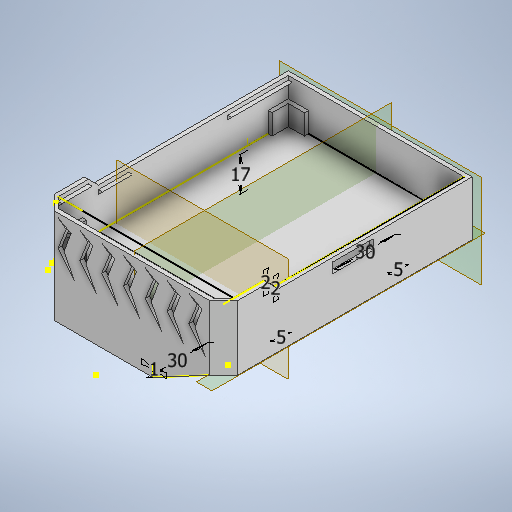
# Autodesk Inventor part: Part1edd
Saved by Autodesk Inventor 2025.2 (Build 292293000, 293)
## iProperties
Created: 2025-06-04
Part Number: Part1edd
Material: Generic
Document SubType Name: Sheet Metal
Designer: ziyuz
Density: 1 g/cm^3
Sheet Metal Rule: Default_mm
Appearance: Default
Author: ziyuz
Autodesk Inventor part; units mm, degrees
ref_plane "YZ Plane" through (0, 0, 0) normal (1, 0, 0) x (0, 1, 0)
ref_plane "XZ Plane" through (0, 0, 0) normal (0, 1, 0) x (-1, 0, 0)
ref_plane "XY Plane" through (0, 0, 0) normal (0, 0, 1) x (1, 0, 0)
sketch "Sketch1" plane through (0, 0, 0) normal (0, 1, 0) x (-1, 0, 0)
  line L0 (0, 0) -> (-85, 0)
  line L1 (-85, 0) -> (-85, -115)
  line L2 (-85, -115) -> (0, -115)
  line L3 (0, -115) -> (0, 0)
  dimension "d0" = 85
  dimension "d1" = 115
  constraints: 8 end point, 2 parallel, 1 horizontal, 1 perpendicular
  measures "d0" distance of L2.end L1.end
  measures "d1" distance of L1.end L0.end
extrude "Extrusion1" add sketch "Sketch1" along normal blind 2
sketch "Sketch2" plane through (0, 2, 0) normal (0, 1, 0) x (1, 0, 0)
  line L0 (0, 115) -> (0, 0) projected
  line L1 (0, 115) -> (-2, 115)
  line L2 (0, 115) -> (0, 117)
  line L3 (0, 117) -> (-2, 117)
  line L4 (-2, 115) -> (-2, 117)
  line L5 (-2, 117) -> (87, 117)
  line L6 (87, 117) -> (87, -2)
  line L7 (87, -2) -> (-2, -2)
  line L8 (-2, -2) -> (-2, 117)
  line L9 (-2, 117) -> (-2, 107)
  line L10 (-2, 107) -> (0, 107)
  line L11 (-2, 117) -> (8, 117)
  line L12 (8, 117) -> (8, 115)
  line L13 (85, 115) -> (0, 115) projected
  line L14 (-2, 115) -> (-2, 5)
  line L15 (-2, 5) -> (-2, 15)
  line L16 (0, 15) -> (0, 5)
  line L17 (8, 5) -> (8, 7)
  line L18 (-2, 5) -> (-2, 3)
  line L19 (-2, 3) -> (10, 3)
  line L20 (10, 3) -> (10, 5)
  line L21 (10, 5) -> (0, 5)
  line L22 (0, 5) -> (0, 15)
  line L23 (0, 15) -> (-2, 15)
  line L24 (-2, 5) -> (-2, 15)
  dimension "d4" = 2
  dimension "d5" = 2
  dimension "d6" = 89
  dimension "d7" = 119
  dimension "d8" = 10
  dimension "d9" = 10
  dimension "d10" = 110
  dimension "d11" = 10
  dimension "d13" = 2
  dimension "d21" = 2
  dimension "d22" = 12
  dimension "d23" = 2
  dimension "d24" = 10
  constraints: 46 end point, 9 point on line, 7 perpendicular, 3 parallel, 2 collinear, 2 horizontal, 1 vertical
  measures "d4" distance of L0.start L1.end
  measures "d5" distance of L0.start L2.end
  measures "d6" distance of L6.end L7.end
  measures "d7" distance of L5.end L6.end
  measures "d8" distance of L3.end L9.end
  measures "d9" distance of L3.end L11.end
  measures "d10" distance of L1.end L14.end
  measures "d11" distance of L14.end L15.end
  measures "d13" distance of L17.start L17.end
  measures "d21" distance of L14.end L18.end
  measures "d22" distance of L18.end L19.end
  measures "d23" distance of L19.end L20.end
  measures "d24" distance of L16.end L16.start
extrude "Extrusion2" add sketch "Sketch2" along normal blind 10 contours L0 L10 L8 L1 | L1 L4 L3 L2 | L2 L5 L12 L13 | L0 L19 L8 L23 | L21 L20 L19 L0
sketch "Sketch3" plane through (0, 2, 0) normal (0, -1, 0) x (1, 0, 0)
  line L0 (8, -117) -> (-2, -117) projected
  line L1 (-2, -117) -> (85, -117)
  line L2 (85, -117) -> (85, 2)
  line L3 (85, 2) -> (-2, 2)
  line L4 (-2, 2) -> (-2, -117)
  point P0 (0, 0)
  point P1 (87, -117)
  dimension "d16" = 87
  dimension "d17" = 119
  constraints: 8 end point, 2 parallel, 1 horizontal, 1 perpendicular
  measures "d16" distance of L3.end L2.end
  measures "d17" distance of L2.end L1.end
extrude "Extrusion3" add sketch "Sketch3" along normal blind 2
sketch "Sketch5" plane through (0, 2, 0) normal (0, 1, 0) x (1, 0, 0)
  line L0 (0, 5) -> (0, 15) projected
  line L1 (85, 117) -> (85, -2) projected
  line L2 (0, 5) -> (85, 5)
  line L3 (85, 5) -> (85, 115)
  line L4 (85, 115) -> (0, 115)
  line L5 (0, 115) -> (0, 5)
  line L6 (0, 5) -> (40, 5)
  line L7 (85, 5) -> (50, 5)
  line L8 (85, -2) -> (-2, -2) projected
  line L9 (40, 5) -> (50, 5)
  line L10 (50, 5) -> (50, -2)
  line L11 (50, -2) -> (40, -2)
  line L12 (40, -2) -> (40, 5)
  point P0 (0, 0)
  dimension "d25" = 110
  dimension "d26" = 40
  dimension "d27" = 35
  constraints: 20 end point, 4 parallel, 4 point on line, 2 horizontal, 2 perpendicular
  measures "d25" distance of L3.end L2.end
  measures "d26" distance of L0.start L6.end
  measures "d27" distance of L2.end L7.end
extrude "Extrusion4" cut sketch "Sketch5" against normal blind 10 contours L2 L10 L8 L12
sketch "Sketch6" plane through (0, 0, 0) normal (0, -1, 0) x (1, 0, 0)
  line L0 (-2, 2) -> (-2, -3) projected
  line L1 (-2, 2) -> (-4, 2)
  line L2 (-4, 2) -> (-4, 4)
  line L3 (-4, 4) -> (-2, 4)
  line L4 (-2, 4) -> (-2, 2)
  line L5 (-4, 4) -> (87, 4)
  line L6 (87, 4) -> (87, -119)
  line L7 (87, -119) -> (-4, -119)
  line L8 (-4, -119) -> (-4, 4)
  line L9 (85, -117) -> (85, 2) projected
  line L10 (-2, 2) -> (85, 2)
  line L11 (85, 2) -> (85, -117)
  line L12 (85, -117) -> (-2, -117)
  line L13 (-2, -117) -> (-2, 2)
  line L14 (-2, -3) -> (-4, -3)
  line L15 (-4, -3) -> (-4, 4)
  line L16 (-4, 4) -> (3, 4)
  line L17 (3, 4) -> (3, 2)
  line L18 (-2, -3) -> (3, 2)
  line L19 (85, -3) -> (85, 2)
  line L20 (85, 2) -> (80, 2)
  line L21 (80, 2) -> (85, -3)
  line L22 (87, -3) -> (85, -3)
  line L23 (80, 2) -> (80, 4)
  line L24 (-4, -3) -> (3, 4)
  line L25 (3, 2) -> (-2, -3)
  line L26 (87, -3) -> (80, 4)
  point P0 (0, 0)
  point P1 (85, 2)
  point P2 (-2, -3)
  point P3 (-2, -3)
  dimension "d30" = 2
  dimension "d31" = 2
  dimension "d32" = 91
  dimension "d33" = 123
  dimension "d36" = 7
  dimension "d37" = 5
  constraints: 50 end point, 8 point on line, 7 parallel, 6 perpendicular, 3 horizontal, 2 collinear
  measures "d30" distance of L2.end L3.end
  measures "d31" distance of L1.end L2.end
  measures "d32" distance of L6.end L7.end
  measures "d33" distance of L5.end L6.end
  measures "d36" distance of L2.end L16.end
  measures "d37" distance of L10.end L20.end
extrude "Extrusion5" add sketch "Sketch6" against normal blind 22 contours L24 L10 L18 L0 | L0 L14 L24 | L24 L17 L10 | L13 L12 L9 L22 L6 L7 L8 L14 | L5 L23 L10 L17 | L26 L10 L23 | L10 L26 L9 L21 | L9 L26 L22
sketch "Sketch7" plane through (0, 2, 0) normal (0, 1, 0) x (1, 0, 0)
  line L0 (-2, -2) -> (-2, 1) projected
  line L1 (-2, -2) -> (-2, 1)
  line L2 (1, -2) -> (-2, -2) projected
  line L3 (1, -2) -> (-2, 1)
  line L4 (-2, -2) -> (1, -2)
  line L5 (85, 1) -> (85, -2) projected
  line L6 (85, -2) -> (85, 1)
  line L7 (85, -2) -> (82, -2)
  line L8 (80, -4) -> (87, 3) projected
  line L9 (85, 1) -> (82, -2)
  point P0 (0, 0)
  constraints: 12 end point, 2 collinear, 2 point on line, 2 vertical
extrude "Extrusion6" cut sketch "Sketch7" against normal blind 22
sketch "Sketch8" plane through (0, 22, 0) normal (0, 1, 0) x (1, 0, 0)
  line L0 (-4, 3) -> (-4, 23)
  line L1 (-4, 3) -> (-4, 119) projected
  line L2 (-4, 23) -> (-2, 23)
  line L3 (-2, 3) -> (-2, 117) projected
  line L4 (-2, 3) -> (3, -2) projected
  line L5 (-2, 3) -> (3, -2)
  line L6 (85, 3) -> (80, -2) projected
  line L7 (3, -2) -> (80, -2)
  line L8 (80, -2) -> (85, 3)
  line L9 (85, 117) -> (85, 3) projected
  line L10 (85, 3) -> (85, 23)
  line L11 (85, 23) -> (87, 23)
  line L12 (87, 119) -> (87, 3) projected
  line L13 (80, -4) -> (87, 3) projected
  line L14 (87, 3) -> (87, 23)
  line L15 (87, 3) -> (80, -4)
  line L16 (-4, 3) -> (3, -4) projected
  line L17 (80, -4) -> (3, -4)
  line L18 (3, -4) -> (-4, 3)
  point P0 (0, 0)
  dimension "d40" = 20
  dimension "d41" = 20
  constraints: 22 end point, 5 point on line, 3 collinear, 2 parallel, 2 perpendicular
  measures "d40" distance of L0.start L0.end
  measures "d41" distance of L6.start L10.end
extrude "Extrusion7" add sketch "Sketch8" along normal blind 5
chamfer "Chamfer1" distance 5 angle 45 2 edges at (86, 27, -23) (-3, 27, -23)
sketch "Sketch9" plane through (3, 0, 4) normal (0, 0, 1) x (1, 0, 0)
  line L0 (0, 2) -> (0, 27) projected
  line L1 (0, 27) -> (0, 25)
  line L2 (0, 2) -> (0, 25)
  line L3 (0, 25) -> (77, 25)
  line L4 (0, 27) -> (77, 27) projected
  line L5 (77, 2) -> (77, 27) projected
  line L6 (77, 25) -> (77, 2)
  line L7 (0, 2) -> (77, 2)
  line L8 (0, 2) -> (2, 2)
  line L9 (5, 2) -> (-3, 2) projected
  line L10 (2, 2) -> (2, 25)
  line L11 (77, 25) -> (75, 25)
  line L12 (75, 25) -> (75, 2)
  line L13 (2, 25) -> (6, 22)
  line L14 (-5, 22) -> (82, 22) projected
  line L15 (6, 22) -> (2, 12)
  line L16 (7, 12) -> (-3, 12) projected
  line L17 (0, 2) -> (10, 2)
  line L18 (5, 2) -> (82, 2) projected
  line L19 (10, 2) -> (10, 25)
  line L20 (2, 12) -> (10, 2)
  line L21 (10, 2) -> (5, 12)
  line L22 (5, 12) -> (8.4202, 21.3969)
  line L23 (5, 12) -> (15, 12) construction
  line L24 (2, 25) -> (8.4202, 21.3969)
  line L25 (12.8, 12) -> (20.8, 2)
  line L26 (20.8, 2) -> (15.8, 12)
  line L27 (15.8, 12) -> (19.2202, 21.3969)
  line L28 (16.8, 22) -> (12.8, 12)
  line L29 (12.8, 25) -> (16.8, 22)
  line L30 (12.8, 25) -> (19.2202, 21.3969)
  line L31 (23.6, 12) -> (31.6, 2)
  line L32 (31.6, 2) -> (26.6, 12)
  line L33 (26.6, 12) -> (30.0202, 21.3969)
  line L34 (27.6, 22) -> (23.6, 12)
  line L35 (23.6, 25) -> (27.6, 22)
  line L36 (23.6, 25) -> (30.0202, 21.3969)
  line L37 (34.4, 12) -> (42.4, 2)
  line L38 (42.4, 2) -> (37.4, 12)
  line L39 (37.4, 12) -> (40.8202, 21.3969)
  line L40 (38.4, 22) -> (34.4, 12)
  line L41 (34.4, 25) -> (38.4, 22)
  line L42 (34.4, 25) -> (40.8202, 21.3969)
  line L43 (45.2, 12) -> (53.2, 2)
  line L44 (53.2, 2) -> (48.2, 12)
  line L45 (48.2, 12) -> (51.6202, 21.3969)
  line L46 (49.2, 22) -> (45.2, 12)
  line L47 (45.2, 25) -> (49.2, 22)
  line L48 (45.2, 25) -> (51.6202, 21.3969)
  line L49 (56, 12) -> (64, 2)
  line L50 (64, 2) -> (59, 12)
  line L51 (59, 12) -> (62.4202, 21.3969)
  line L52 (60, 22) -> (56, 12)
  line L53 (56, 25) -> (60, 22)
  line L54 (56, 25) -> (62.4202, 21.3969)
  line L55 (66.8, 12) -> (74.8, 2)
  line L56 (74.8, 2) -> (69.8, 12)
  line L57 (69.8, 12) -> (73.2202, 21.3969)
  line L58 (70.8, 22) -> (66.8, 12)
  line L59 (66.8, 25) -> (70.8, 22)
  line L60 (66.8, 25) -> (73.2202, 21.3969)
  point P0 (-3, 0)
  dimension "d47" = 2
  dimension "d48" = 2
  dimension "d49" = 2
  dimension "d50" = 5
  dimension "d51" = 10
  dimension "d52" = 10
  dimension "d53" = 70
  dimension "d56" = 10.8
  constraints: 108 end point, 9 point on line, 4 perpendicular, 2 collinear, 2 horizontal, 1 equal length, 1 midpoint, 1 parallel, 72 other
  measures "d47" distance of L0.end L1.end
  measures "d48" distance of L0.start L8.end
  measures "d49" distance of L3.end L11.end
  measures "d50" distance of L10.end L13.end
  measures "d51" distance of L0.start L17.end
  measures "d52" distance of L21.end L22.end
  measures "d53" angle of L23 L22
  measures "d56" distance of L15.end L25.start
extrude "Extrusion8" cut sketch "Sketch9" against normal blind 5 contours L24 L14 L13 | L14 L24 L22 L16 L15 | L16 L21 L20 | L30 L14 L29 | L36 L14 L35 | L14 L30 L27 L26 L25 L28 | L60 L14 L59 | L42 L14 L41 | L14 L36 L33 L32 L31 L34 | L54 L14 L53 | L14 L60 L57 L56 L55 L58 | L48 L14 L47 | L14 L42 L39 L38 L37 L40 | L14 L54 L51 L50 L49 L52 | L14 L48 L45 L44 L43 L46
sketch "Sketch10" plane through (87, 0, -3) normal (1, 0, 0) x (0, 0, -1)
  line L0 (112, 2) -> (112, 12) projected
  line L1 (112, 2) -> (2, 2)
  line L2 (114, 12) -> (104, 12) projected
  line L3 (112, 2) -> (222, 2) construction
  line L4 (12, 2) -> (104, 2) projected
  line L5 (0, 0) -> (116, 0) projected
  line L6 (112, 2) -> (112, 20)
  line L7 (112, 20) -> (67, 20)
  line L8 (67, 20) -> (67, 15)
  line L9 (2, 2) -> (2, 20)
  line L10 (2, 20) -> (47, 20)
  line L11 (47, 20) -> (47, 15)
  line L12 (67, 15) -> (47, 15)
  line L13 (47, 20) -> (67, 20)
  point P0 (-3, 0)
  dimension "d63" = 110
  dimension "d64" = 180
  dimension "d67" = 18
  dimension "d68" = 45
  dimension "d69" = 18
  dimension "d70" = 45
  constraints: 20 end point, 5 perpendicular, 2 parallel, 2 point on line, 1 collinear, 1 horizontal
  measures "d63" distance of L0.start L1.end
  measures "d64" angle of L1 L3
  measures "d67" distance of L0.start L6.end
  measures "d68" distance of L6.end L7.end
  measures "d69" distance of L1.end L9.end
  measures "d70" distance of L9.end L10.end
extrude "Extrusion9" cut sketch "Sketch10" against normal blind 10 contours L8 L12 L11 L13
sketch "Sketch11" plane through (0, 2, 0) normal (0, 1, 0) x (1, 0, 0)
  line L0 (-2, 23) -> (-2, 117) projected
  line L1 (85, 23) -> (85, 18) projected
  line L2 (-2, 117) -> (85, 117)
  line L3 (85, 117) -> (85, 23)
  line L4 (85, 23) -> (-2, 23)
  line L5 (-2, 23) -> (-2, 117)
  point P0 (0, 0)
  constraints: 8 end point, 2 parallel, 1 horizontal, 1 perpendicular
sketch "Sketch12" plane through (85, 2, -117) normal (-1, 0, 0) x (0, 0, 1)
  line L0 (0, 0) -> (0, 20) projected
  line L1 (0, 20) -> (94, 20) projected
  line L2 (0, 20) -> (94, 20)
  line L3 (99, 25) -> (114, 25) projected
  line L4 (94, 20) -> (99, 25)
  line L5 (114, 25) -> (119, 25) projected
  line L6 (114, 25) -> (99, 25)
  line L7 (99, 25) -> (99, 23)
  line L8 (94, 20) -> (94, 18)
  point P0 (117, -2)
  dimension "d73" = 2
  dimension "d74" = 2
  constraints: 10 end point, 2 vertical, 1 horizontal, 1 parallel
  measures "d73" distance of L3.start L7.end
  measures "d74" distance of L1.end L8.end
sketch "Sketch13" plane through (0, 27, 0) normal (0, 1, 0) x (1, 0, 0)
  line L0 (85, 18) -> (85, 3) projected
  line L1 (-2, 3) -> (10, 3) projected
  line L2 (85, 3) -> (-2, 3)
  point P0 (0, 0)
  constraints: 2 end point, 1 horizontal
sketch "Sketch14" plane through (85, 2, -117) normal (-1, 0, 0) x (0, 0, 1)
  line L0 (114, 25) -> (99, 25) projected
  line L1 (99, 25) -> (99, 23)
  line L2 (99, 23) -> (114, 23)
  line L3 (99, 23) -> (99, 21)
  line L4 (99, 21) -> (114, 21)
  line L5 (114, 0) -> (114, 25) projected
  line L6 (114, 23) -> (114, 21)
  line L7 (94, 20) -> (99, 25) projected
  line L8 (94, 20) -> (94, 18)
  line L9 (94, 18) -> (79, 18)
  line L10 (79, 18) -> (79, 20)
  line L11 (0, 20) -> (94, 20) projected
  line L12 (94, 18) -> (94, 16)
  line L13 (94, 16) -> (79, 16)
  line L14 (79, 18) -> (79, 16)
  line L15 (0, 20) -> (0, 18)
  line L16 (0, 0) -> (0, 20) projected
  line L17 (0, 18) -> (30, 18)
  line L18 (30, 18) -> (30, 20)
  line L19 (0, 18) -> (30, 18)
  line L20 (30, 18) -> (30, 16)
  line L21 (30, 16) -> (0, 16)
  line L22 (0, 16) -> (0, 18)
  point P0 (117, -2)
  dimension "d75" = 2
  dimension "d76" = 2
  dimension "d77" = 2
  dimension "d78" = 15
  dimension "d79" = 2
  dimension "d80" = 2
  dimension "d81" = 30
  dimension "d82" = 90
  dimension "d83" = 2
  constraints: 36 end point, 10 perpendicular, 5 point on line, 3 vertical, 2 parallel, 1 horizontal
  measures "d75" distance of L0.end L1.end
  measures "d76" distance of L1.end L3.end
  measures "d77" distance of L7.start L8.end
  measures "d78" distance of L8.end L9.end
  measures "d79" distance of L8.end L12.end
  measures "d80" distance of L11.start L15.end
  measures "d81" distance of L15.end L17.end
  measures "d82" angle of L17 L15
  measures "d83" distance of L19.end L20.end
extrude "Extrusion10" add sketch "Sketch14" along normal blind 2 contours L5 L4 L3 L2 | L12 L13 L14 L9 | L17 L20 L21 L16
chamfer "Chamfer2" distance 2 angle 45 3 edges at (83, 18, -102) (83, 18, -30.5) (83, 23, -10.5)
sketch "Sketch15" plane through (0, 2, 0) normal (0, 1, 0) x (1, 0, 0)
  point P0 (0, 0)
ref_plane "Work Plane1" through (41.5, 0, -119) normal (-1, 0, 0) x (0, 0, 1)
mirror "Mirror1" about plane through (41.5, 0, -119) normal (-1, 0, 0) of "Extrusion10"
chamfer "Chamfer3" distance 2 angle 45 3 edges at (0, 23, -10.5) (0, 18, -30.5) (0, 18, -102)
sketch "Sketch16" plane through (0, 0, 0) normal (0, -1, 0) x (1, 0, 0)
  line L0 (50, -5) -> (50, 2) projected
  line L1 (50, 2) -> (50, 4)
  line L2 (3, 4) -> (80, 4) projected
  line L3 (50, 4) -> (52, 4)
  line L4 (52, 4) -> (52, -119)
  line L5 (87, -119) -> (-4, -119) projected
  line L6 (52, -119) -> (-4, -119)
  line L7 (3, 4) -> (-4, -3) projected
  line L8 (-4, -119) -> (-4, -3)
  line L9 (-4, -3) -> (3, 4)
  line L10 (3, 4) -> (52, 4)
  line L11 (50, 2) -> (50, -117)
  line L12 (-2, -117) -> (-2, -107) projected
  line L13 (50, -117) -> (-2, -117)
  line L14 (-2, -3) -> (0, -3) projected
  line L15 (-2, -117) -> (-2, -3)
  line L16 (80, 2) -> (3, 2) projected
  line L17 (-2, -3) -> (3, 2)
  point P0 (0, 0)
  dimension "d93" = 2
  dimension "d94" = 90
  dimension "d95" = 119
  dimension "d96" = 52
  constraints: 22 end point, 4 point on line, 3 collinear, 1 parallel, 1 perpendicular, 1 vertical
  measures "d93" distance of L1.end L3.end
  measures "d94" angle of L3 L4
  measures "d95" distance of L0.end L11.end
  measures "d96" distance of L11.end L12.start
extrude "Extrusion11" add sketch "Sketch16" along normal blind 20
sketch "Sketch17" plane through (-2, 0, -3) normal (1, 0, 0) x (0, 0, -1)
  point P0 (-3, 0)
sketch "Sketch18" plane through (0, 0, 0) normal (0, -1, 0) x (1, 0, 0)
  line L0 (-2, -3) -> (-2, -117) projected
  line L1 (-2, -117) -> (-2, -7)
  line L2 (-2, -7) -> (28, -7)
  line L3 (28, -7) -> (28, -117)
  line L4 (28, -117) -> (-2, -117)
  line L5 (-2, -117) -> (-2, -97)
  line L6 (-2, -15) -> (-2, -107) projected
  line L7 (-2, -97) -> (28, -97)
  line L8 (-2, -7) -> (-2, -27)
  line L9 (-2, -27) -> (28, -27)
  line L10 (28, -7) -> (28, 2)
  line L11 (80, 2) -> (3, 2) projected
  line L12 (28, -7) -> (30, -7)
  line L13 (30, -7) -> (30, -117)
  line L14 (-2, -117) -> (85, -117) projected
  line L15 (28, -117) -> (30, -117)
  line L16 (-2, -97) -> (-2, -99)
  line L17 (-2, -99) -> (28, -99)
  line L18 (-2, -27) -> (-2, -25)
  line L19 (-2, -25) -> (28, -25)
  line L20 (30, -7) -> (50, -7)
  line L21 (50, -117) -> (50, -5) projected
  line L22 (50, -5) -> (40, -5) projected
  line L23 (50, -5) -> (28, -5)
  line L24 (30, -7) -> (30, -62)
  line L25 (30, -62) -> (50, -62)
  line L26 (30, -62) -> (30, -61)
  line L27 (30, -61) -> (50, -61)
  line L28 (30, -62) -> (30, -63)
  line L29 (30, -63) -> (50, -63)
  point P0 (0, 0)
  dimension "d99" = 110
  dimension "d100" = 30
  dimension "d101" = 20
  dimension "d102" = 20
  dimension "d103" = 2
  dimension "d104" = 2
  dimension "d105" = 2
  dimension "d106" = 1
  dimension "d107" = 1
  constraints: 48 end point, 16 point on line, 10 perpendicular, 4 horizontal, 2 midpoint, 1 vertical
  measures "d99" distance of L0.end L1.end
  measures "d100" distance of L1.end L2.end
  measures "d101" distance of L0.end L5.end
  measures "d102" distance of L1.end L8.end
  measures "d103" distance of L2.end L12.end
  measures "d104" distance of L5.end L16.end
  measures "d105" distance of L8.end L18.end
  measures "d106" distance of L24.end L26.end
  measures "d107" distance of L24.end L28.end
extrude "Extrusion12" add sketch "Sketch18" along normal blind 17 contours L12 L13 L14 L3 | L10 L23 L22 L21 L20 L12 | L19 L3 L9 L0 | L27 L21 L25 L13 | L7 L3 L17 L0 | L25 L21 L29 L13
sketch "Sketch19" plane through (-2, -20, -3) normal (1, 0, 0) x (0, 0, -1)
  line L0 (94, 20) -> (94, 3)
  line L1 (94, 3) -> (94, 20) projected
  line L2 (94, 3) -> (24, 3)
  line L3 (24, 20) -> (24, 3) projected
  point P0 (-3, 20)
  dimension "d110" = 17
  constraints: 4 end point, 2 point on line, 1 perpendicular
  measures "d110" distance of L0.start L0.end
sketch "Sketch20" plane through (-2, 0, -25) normal (0, 0, 1) x (1, 0, 0)
  line L0 (0, -17) -> (0, 0) projected
  line L1 (0, -17) -> (10, -17)
  line L2 (30, -17) -> (0, -17) projected
  line L3 (10, -17) -> (20, -17)
  line L4 (20, -17) -> (20, 0)
  line L5 (0, 0) -> (30, 0) projected
  line L6 (20, 0) -> (10, 0)
  line L7 (10, 0) -> (9.6696, 0.5865)
  line L8 (10, -17) -> (10, 0)
  line L9 (10, 0) -> (10, -5)
  line L10 (10, -5) -> (20, -5)
  line L11 (10, -17) -> (10, -12)
  line L12 (10, -12) -> (20, -12)
  point P0 (2, 0)
  dimension "d111" = 10
  dimension "d112" = 10
  dimension "d113" = 90
  dimension "d114" = 5
  dimension "d115" = 5
  constraints: 20 end point, 7 point on line, 4 perpendicular
  measures "d111" distance of L0.start L1.end
  measures "d112" distance of L1.end L3.end
  measures "d113" angle of L4 L3
  measures "d114" distance of L6.end L9.end
  measures "d115" distance of L1.end L11.end
extrude "Extrusion13" cut sketch "Sketch20" against normal blind 17 contours L8 L10 L4 L12
ref_plane "Work Plane2" through (87, 22, -119) normal (0, 0, -1) x (-1, 0, 0)
sketch "Sketch21" plane through (87, 22, -119) normal (0, 0, -1) x (-1, 0, 0)
  line L0 (0, -22) -> (7, -22) projected
  line L1 (7, -22) -> (7, -27)
  line L2 (35, -22) -> (35, -42) projected
  line L3 (7, -27) -> (35, -42)
  line L4 (7, -27) -> (0, -27)
  line L5 (0, -22) -> (0, -27)
  line L6 (35, -42) -> (35, -22)
  line L7 (35, -22) -> (7, -22)
  point P0 (87, -22)
  dimension "d119" = 5
  constraints: 12 end point, 2 perpendicular, 1 collinear, 1 horizontal, 1 vertical
  measures "d119" distance of L0.end L1.end
extrude "Extrusion14" add sketch "Sketch21" against normal blind 116
sketch "Sketch22" plane through (87, 22, -3) normal (0, 0, 1) x (1, 0, 0)
  line L0 (-7, -22) -> (-35, -22) projected
  line L1 (-7, -27) -> (-35, -42) projected
  line L2 (-7, -22) -> (-7, -27)
  line L3 (-35, -42) -> (-84, -42) projected
  line L4 (-7, -27) -> (-35, -42)
  line L5 (-7, -22) -> (-35, -22)
  line L6 (-35, -22) -> (-35, -42)
  point P0 (-87, -22)
  constraints: 8 end point, 1 horizontal, 1 perpendicular, 1 vertical
extrude "Extrusion15" add sketch "Sketch22" along normal blind 7
sketch "Sketch23" plane through (0, 0, 0) normal (0, -1, 0) x (1, 0, 0)
  line L0 (80, 4) -> (87, -3) projected
  line L1 (80, -3) -> (87, -3) projected
  line L2 (87, -3) -> (80, -3)
  line L3 (3, 4) -> (80, 4) projected
  line L4 (80, -3) -> (80, 4)
  line L5 (80, 4) -> (87, -3)
  point P0 (0, 0)
  constraints: 6 end point, 1 collinear, 1 perpendicular
extrude "Extrusion16" add sketch "Sketch23" along normal blind 5
ref_plane "Work Plane3" through (80, -5, -119) normal (0, -1, 0) x (1, 0, 0)
sketch "Sketch24" plane through (80, -5, -119) normal (0.4722214, -0.88148, 0) x (0.88148, 0.4722214, 0)
  line L0 (0, 0) -> (-31.7648, 0) projected
  line L1 (-31.7648, 123) -> (0, 123) projected
  line L2 (-31.7648, 0) -> (-31.7648, 123)
  line L3 (-31.7648, 123) -> (-31.7648, 93)
  line L4 (-31.7648, 93) -> (0, 93)
  line L5 (0, 93) -> (0, 88)
  line L6 (0, 88) -> (-31.7648, 88)
  line L7 (-31.7648, 0) -> (-31.7648, 30)
  line L8 (-31.7648, 0) -> (-31.7648, 123) projected
  line L9 (-31.7648, 30) -> (0, 30)
  line L10 (0, 30) -> (0, 35)
  line L11 (0, 35) -> (-31.7648, 35)
  line L12 (-31.7648, 35) -> (-31.7648, 30)
  point P0 (-68.1573, 119)
  dimension "d127" = 30
  dimension "d128" = 5
  dimension "d129" = 30
  dimension "d130" = 5
  constraints: 20 end point, 6 perpendicular, 6 point on line, 1 collinear
  measures "d127" distance of L1.start L3.end
  measures "d128" distance of L4.end L5.end
  measures "d129" distance of L0.end L7.end
  measures "d130" distance of L9.end L10.end
ref_plane "Work Plane4" through (3, 27, -31) normal (0, 0, 1) x (1, 0, 0)
sketch "Sketch25" plane through (3, 27, -31) normal (0, 0, 1) x (1, 0, 0)
  line L0 (77, -32) -> (49, -47)
  line L1 (77, -32) -> (77, 0) projected
  line L2 (77, -32) -> (49, -47)
  line L3 (49, -47) -> (49, -41.7688)
  line L4 (77, -32) -> (77, -30)
  line L5 (49, -41.7688) -> (77, -30)
  line L6 (77, -30) -> (77, -32)
  line L7 (77, -30) -> (77, -33)
  line L8 (77, -33) -> (49, -47)
  point P0 (-3, -27)
  dimension "d133" = 2
  dimension "d134" = 3
  constraints: 16 end point, 2 collinear, 2 point on line, 1 vertical
  measures "d133" distance of L0.start L4.end
  measures "d134" distance of L4.end L7.end
extrude "Extrusion17" cut sketch "Sketch25" along normal blind 5
pattern_linear "Rectangular Pattern1" count 2 spacing 58 along (0, 0, -1) of "Extrusion17"
sketch "Sketch26" plane through (3, 27, 4) normal (0, 0, 1) x (1, 0, 0)
  line L0 (49, -41.7688) -> (49, -47) projected
  line L1 (49, -44.3844) -> (50, -44.3844)
  point P0 (-3, -27)
  dimension "d140" = 1
  constraints: 2 end point, 1 horizontal, 1 midpoint
  measures "d140" distance of L1.start L1.end
sketch "Sketch27" plane through (3, 27, -31) normal (0, 0, 1) x (1, 0, 0)
  line L0 (77, -30) -> (49, -41.7688) projected
  line L1 (49, -41.7688) -> (51.7656, -40.6064)
  line L2 (49, -41.7688) -> (49, -43.7688)
  line L3 (49, -41.7688) -> (49, -47) projected
  line L4 (49, -43.7688) -> (51.7656, -42.6064)
  circle A0 centre (51.7656, -42.6064) radius 1
  point P0 (-3, -27)
  dimension "d141" = 3
  dimension "d142" = 2
  dimension "d143" = 3
  dimension "d144" = 2
  constraints: 6 end point, 2 point on line, 1 centre point, 1 coincident
  measures "d141" distance of L0.end L1.end
  measures "d142" distance of L0.end L2.end
  measures "d143" distance of L2.end L4.end
  measures "d144" diameter of A0
extrude "Extrusion18" cut sketch "Sketch27" along normal blind 5.1 and the other way blind 0.1
pattern_linear "Rectangular Pattern2" count 2 spacing 58 along (0, 0, -1) of "Extrusion18"
equation "\"BendRadius\" = Thickness"
equation "\"BendReliefWidth\" = Thickness"
equation "\"BendReliefDepth\" = 0.5 * Thickness"
equation "\"CornerReliefSize\" = 4 * Thickness"
equation "\"MinimumRemnant\" = 2 * Thickness"
equation "\"TransitionRadius\" = BendRadius"
equation "\"JacobiRadiusSize\" = BendRadius"
equation "\"GapSize\" = Thickness"
equation "\"Thickness\" = 0.5"
body "Solid1"
